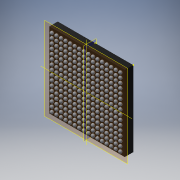
# Autodesk Inventor part: SiP
Saved by Autodesk Inventor 2017 (Build 210142000, 142)
## iProperties
Created: 2018-07-04
Part Number: SiP
Material: Generic
Document SubType Name: Modeling
Designer: intelsath
Density: 1 g/cm^3
Appearance: Default
Author: intelsath
Autodesk Inventor part; units mm, degrees
ref_plane "YZ Plane" through (0, 0, 0) normal (1, 0, 0) x (0, 1, 0)
ref_plane "XZ Plane" through (0, 0, 0) normal (0, 1, 0) x (-1, 0, 0)
ref_plane "XY Plane" through (0, 0, 0) normal (0, 0, 1) x (1, 0, 0)
sketch "Sketch1" plane through (0, 0, 0) normal (0, 1, 0) x (-1, 0, 0)
  line L0 (0, 0) -> (21, 0)
  line L1 (21, 0) -> (21, -21)
  line L2 (21, -21) -> (0, -21)
  line L3 (0, -21) -> (0, 0)
  dimension "d0" = 21
  dimension "d1" = 21
  constraints: 8 end point, 2 parallel, 1 horizontal, 1 perpendicular
  measures "d0" distance of L1.end L2.end
  measures "d1" distance of L0.end L1.end
extrude "Extrusion1" add sketch "Sketch1" along normal blind 2.35
ref_plane "Work Plane1" through (0, -0.25, 0) normal (0, -1, 0) x (1, 0, 0)
sketch "Sketch2" plane through (0, -0.25, 0) normal (0, -1, 0) x (1, 0, 0)
  line L0 (0, 0) -> (0, -21) construction
  line L1 (0, -10.5) -> (-21, -10.5) construction
  line L2 (-21, -21) -> (-21, 0) construction
  line L3 (-10.5, -10.5) -> (-10.5, 0) construction
  circle A0 centre (-9.865, -9.865) radius 0.45
  line L4 (-10.264, -10.0732) -> (-9.466, -9.6568)
  dimension "d9" = 0.635
  dimension "d10" = 0.635
  dimension "d11" = 0.9
  constraints: 6 end point, 4 midpoint, 2 point on circle, 1 centre point, 1 coincident, 1 vertical
  measures "d9" distance from line of L3 point (-9.865, -9.865)
  measures "d10" distance from line of point (-9.865, -9.865) L1
  measures "d11" diameter of A0
revolve "Revolution1" add sketch "Sketch2" angle 360 about axis through (-10.264, -0.25, -10.0732) along (0.8865743, 0, 0.4625862) picked at (-9.8264, -10.0899) contours A0 L4
pattern_linear "Rectangular Pattern1" count 8 spacing 1.27 along (1, 0, 0) count 8 spacing 1.27 along (0, 0, 1) of "Revolution1"
pattern_linear "Rectangular Pattern2" count 2 spacing 10.16 along (0, 0, -1) count 2 spacing 10.16 along (-1, 0, 0) of "Revolution1", "Rectangular Pattern1"
sketch "Sketch3" plane through (0, 2.35, 0) normal (0, 1, 0) x (1, 0, 0)
  line L0 (-19.2325, 16.0212) -> (-2.3216, 16.0212) construction
  line L1 (-2.3216, 16.0212) -> (-2.3216, 6.7909) construction
  line L2 (-2.3216, 6.7909) -> (-19.2325, 6.7909) construction
  line L3 (-19.2325, 6.7909) -> (-19.2325, 16.0212) construction
  line L4 (-20.4185, 17.768) -> (-15.4137, 17.768) construction
  line L5 (-15.4137, 17.768) -> (-15.4137, 12.8722) construction
  line L6 (-15.4137, 12.8722) -> (-20.4185, 12.8722) construction
  line L7 (-20.4185, 12.8722) -> (-20.4185, 17.768) construction
  point P0 (0, 0)
  dimension "d3" = 0
  constraints: 4 other
ref_plane "Work Plane2" through (-10.5, 2.35, 0) normal (-1, 0, 0) x (0, 0, 1)
body "Solid1"
